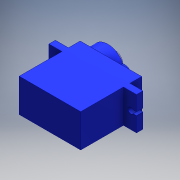
# Autodesk Inventor part: micro-servo
Saved by Autodesk Inventor 2016 (Build 200138000, 138)
## iProperties
Created: 2016-01-12
Part Number: micro-servo
Material: Generic
Document SubType Name: Modeling
Designer: jferner
Density: 1 g/cm^3
Appearance: Default
Author: jferner
Autodesk Inventor part; units mm, degrees
ref_plane "YZ Plane" through (0, 0, 0) normal (1, 0, 0) x (0, 1, 0)
ref_plane "XZ Plane" through (0, 0, 0) normal (0, 1, 0) x (-1, 0, 0)
ref_plane "XY Plane" through (0, 0, 0) normal (0, 0, 1) x (1, 0, 0)
sketch "Sketch1" plane through (0, 0, 0) normal (0, 1, 0) x (-1, 0, 0)
  line L0 (0, 0) -> (-22.66, 0)
  line L1 (-22.66, 0) -> (-22.66, -12.25)
  line L2 (-22.66, -12.25) -> (0, -12.25)
  line L3 (0, -12.25) -> (0, 0)
  dimension "innerLength" = 22.66
  dimension "width" = 12.25
  constraints: 8 end point, 2 parallel, 1 horizontal, 1 perpendicular
  measures "innerLength" distance of L1.end L2.end
  measures "width" distance of L0.end L1.end
extrude "Extrusion1" add sketch "Sketch1" along normal blind 22.48
sketch "Sketch2" plane through (0, 0, -12.25) normal (-1, 0, 0) x (0, 0, 1)
  line L0 (0, 0) -> (0, 22.48) projected
  line L1 (0, 18.14) -> (12.25, 18.14)
  line L2 (12.25, 18.14) -> (12.25, 15.76)
  line L3 (12.25, 15.76) -> (0, 15.76)
  line L4 (0, 15.76) -> (0, 18.14)
  line L5 (0, 22.48) -> (12.25, 22.48) projected
  line L6 (12.25, 0) -> (12.25, 22.48) projected
  dimension "lipOffsetFromTop" = 4.34
  dimension "lipHeight" = 2.38
  constraints: 8 end point, 2 parallel, 1 collinear, 1 horizontal, 1 perpendicular, 1 point on line
  measures "lipOffsetFromTop" distance between parallel lines of L5 L1
  measures "lipHeight" distance of L1.end L2.end
extrude "Extrusion2" add sketch "Sketch2" along normal blind 4.82 contours L0 L1 L2 L3
sketch "Sketch3" plane through (22.66, 0, 0) normal (1, 0, 0) x (0, 0, -1)
  line L0 (0, 18.14) -> (12.25, 18.14)
  line L1 (12.25, 18.14) -> (12.25, 15.76)
  line L2 (12.25, 15.76) -> (0, 15.76)
  line L3 (0, 15.76) -> (0, 18.14)
  line L4 (12.25, 0) -> (12.25, 22.48) projected
  line L5 (0, 0) -> (0, 22.48) projected
  line L6 (0, 22.48) -> (12.25, 22.48) projected
  dimension "d8" = 4.34
  dimension "d9" = 2.38
  constraints: 8 end point, 2 collinear, 2 parallel, 1 horizontal, 1 perpendicular
  measures "d8" distance between parallel lines of L6 L0
  measures "d9" distance between parallel lines of L0 L2
extrude "Extrusion3" add sketch "Sketch3" along normal blind 4.82 contours L0 L1 L2 L3
sketch "Sketch4" plane through (0, 22.48, 0) normal (0, 1, 0) x (1, 0, 0)
  arc A0 (11.646, 8.7771) -> (11.646, 3.4729) centre (6.125, 6.125) ccw
  arc A1 (11.646, 3.4729) -> (11.646, 8.7771) centre (12.25, 6.125) ccw
  line L0 (22.66, 12.25) -> (0, 12.25) projected
  line L1 (0, 12.25) -> (0, 0) projected
  line L2 (0, 0) -> (22.66, 0) projected
  dimension "d12" = 5.44
  constraints: 5 point on circle, 3 tangent, 2 centre point, 1 horizontal alignment
  measures "d12" diameter of A1
extrude "Extrusion4" add sketch "Sketch4" along normal blind 4.1 contours A1 A0
sketch "Sketch5" plane through (0, 26.58, 0) normal (0, 1, 0) x (1, 0, 0)
  circle A0 centre (6.125, 6.125) radius 2.435
  arc A1 (11.646, 8.7771) -> (11.646, 3.4729) centre (6.125, 6.125) ccw projected
  point P0 (0, 0)
  dimension "shaftDiameter" = 4.87
  constraints: 1 centre point, 1 concentric
  measures "shaftDiameter" diameter of A0
extrude "Extrusion5" add sketch "Sketch5" along normal blind 2.94
sketch "Sketch6" plane through (22.66, 18.14, 0) normal (0, 1, 0) x (1, 0, 0)
  arc A0 (3.62, 6.725) -> (3.62, 5.525) centre (2.7401, 6.125) ccw
  line L0 (4.82, 0) -> (4.82, 12.25) projected
  line L1 (4.82, 5.525) -> (3.62, 5.525)
  line L2 (4.82, 6.725) -> (3.62, 6.725)
  line L3 (0, 12.25) -> (4.82, 12.25) projected
  point P0 (-22.66, 0)
  dimension "mountingHoleDiameter" = 2.13
  dimension "d19" = 1.2
  dimension "d20" = 1.2
  dimension "d21" = 0.6
  dimension "d22" = 6.125
  dimension "mountingHoleOffset" = 2.0799
  constraints: 4 end point, 2 point on circle, 2 point on line, 1 centre point, 1 parallel, 1 perpendicular
  measures "mountingHoleDiameter" diameter of A0
  measures "d19" distance of L2.start L2.end
  measures "d20" distance between parallel lines of L2 L1
  measures "d21" distance from line of A0.centre L2
  measures "d22" distance from line of L3 A0.centre
  measures "mountingHoleOffset" distance from line of L0 A0.centre
extrude "Extrusion6" cut sketch "Sketch6" against normal through all
sketch "Sketch7" plane through (0, 18.14, 0) normal (0, 1, 0) x (1, 0, 0)
  arc A0 (-3.62, 5.525) -> (-3.62, 6.725) centre (-2.7401, 6.125) ccw
  line L0 (0, 12.25) -> (-4.82, 12.25) projected
  line L1 (-4.82, 5.525) -> (-3.62, 5.525)
  line L2 (-4.82, 6.725) -> (-3.62, 6.725)
  line L3 (-4.82, 0) -> (-4.82, 12.25) projected
  line L4 (-4.82, 6.725) -> (-4.82, 5.525)
  point P0 (0, 0)
  dimension "d27" = 2.13
  dimension "d29" = 6.125
  dimension "d31" = 1.2
  dimension "d32" = 1.2
  dimension "d33" = 0.6
  constraints: 6 end point, 2 point on circle, 1 centre point, 1 horizontal, 1 parallel, 1 point on line, 1 vertical
  measures "d27" diameter of A0
  measures "d29" distance from line of L0 A0.centre
  measures "d31" distance of L1.start L1.end
  measures "d32" distance between parallel lines of L2 L1
  measures "d33" distance from line of A0.centre L2
extrude "Extrusion7" cut sketch "Sketch7" against normal through all
sketch "Sketch8" plane through (0, 0, -12.25) normal (-1, 0, 0) x (0, 0, 1)
  circle A0 centre (5.125, 5) radius 0.5
  circle A1 centre (6.125, 5) radius 0.5
  circle A2 centre (7.125, 5) radius 0.5
  line L0 (0, 0) -> (0, 15.76) projected
  line L1 (2.9548, 5) -> (8.7957, 5)
  line L2 (0, 0) -> (12.25, 0) projected
  dimension "d36" = 1
  dimension "d37" = 6.125
  dimension "d38" = 5
  constraints: 4 equal radius, 3 centre point, 3 point on line, 2 end point, 1 horizontal
  measures "d36" diameter of A0
  measures "d37" distance from line of L0 A1.centre
  measures "d38" distance from line of L2 A1.centre
extrude "Extrusion8" add sketch "Sketch8" along normal blind 2
equation "\"lipLength\" = -0.5 * innerLength + 0.5 * length"
equation "\"d8\" = lipOffsetFromTop"
equation "\"d9\" = lipHeight"
equation "\"d10\" = lipLength"
equation "\"d20\" = d19"
equation "\"d21\" = 0.5 * d19"
equation "\"d22\" = 0.5 * width"
equation "\"d27\" = mountingHoleDiameter"
equation "\"d29\" = 0.5 * width"
equation "\"d31\" = d19"
equation "\"d32\" = d19"
equation "\"d33\" = 0.5 * d19"
equation "\"d37\" = 0.5 * width"
equation "\"length\" = 32.3"
body "Solid1"
